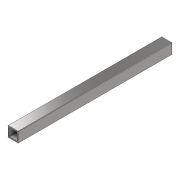
# Autodesk Inventor part: 16x16x2 voor noodstop
Saved by Autodesk Inventor 2020.3 (Build 243373000, 373)
## iProperties
Created: 2020-12-02
Part Number: 16x16x2 voor noodstop
Material: Stainless Steel
Document SubType Name: Modeling
Designer: Svend
Density: 8 g/cm^3
Appearance: Semi-Polished
Author: Svend
Autodesk Inventor part; units mm, degrees
ref_plane "YZ Plane" through (0, 0, 0) normal (1, 0, 0) x (0, 1, 0)
ref_plane "XZ Plane" through (0, 0, 0) normal (0, 1, 0) x (-1, 0, 0)
ref_plane "XY Plane" through (0, 0, 0) normal (0, 0, 1) x (1, 0, 0)
sketch "Sketch1" plane through (0, 0, 0) normal (0, 0, 1) x (1, 0, 0)
  line L0 (-7.5, 7.5) -> (7.5, 7.5)
  line L1 (7.5, 7.5) -> (7.5, -7.5)
  line L2 (7.5, -7.5) -> (-7.5, -7.5)
  line L3 (-7.5, -7.5) -> (-7.5, 7.5)
  line L4 (-7.5, 7.5) -> (7.5, -7.5) construction
  line L5 (7.5, 7.5) -> (-7.5, -7.5) construction
  line L6 (5.5, 5.5) -> (-5.5, 5.5)
  line L7 (-5.5, 5.5) -> (-5.5, -5.5)
  line L8 (-5.5, -5.5) -> (5.5, -5.5)
  line L9 (5.5, -5.5) -> (5.5, 5.5)
  point P0 (0, 0)
  dimension "d0" = 15
  dimension "d1" = 15
  dimension "d2" = 2
  constraints: 20 end point, 4 parallel, 2 midpoint, 2 perpendicular, 1 horizontal, 3 other
  measures "d0" distance of L1.end L2.end
  measures "d1" distance of L0.end L1.end
  measures "d2" distance between parallel lines of L0 L6
extrude "Extrusion1" add sketch "Sketch1" along normal blind 220
fillet "Fillet1" radius 0.5 24 edges at (-5.5, 0, 0) (5.5, 0, 0) (0, -5.5, 0) (0, 5.5, 0) (0, -7.5, 0) (0, 7.5, 0) (-7.5, 7.5, 110) (-7.5, -7.5, 110) (-5.5, 0, 220) (-5.5, -5.5, 110) (-5.5, 5.5, 110) (0, -5.5, 220) (0, 5.5, 220) (0, -7.5, 220) (0, 7.5, 220) (5.5, 0, 220) (5.5, -5.5, 110) (5.5, 5.5, 110) (7.5, 0, 220) (7.5, -7.5, 110) (7.5, 7.5, 110) (7.5, 0, 0) (-7.5, 0, 0) (-7.5, 0, 220)
equation "\"d1\" = d0"
body "Solid1"
